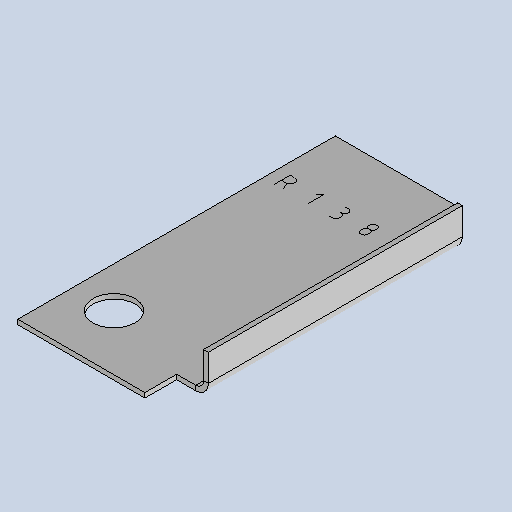
# Autodesk Inventor part: Part14
Saved by Autodesk Inventor 2025.3 (Build 293356030, 356C)
## iProperties
Created: 2026-01-14
Part Number: Part14
Material: Stainless Steel
Document SubType Name: Sheet Metal
Designer: admin
Mass: 447.548 g
Surface Area: 393.455 cm^2
Volume: 55.9434 cm^3
Density: 8 g/cm^3
Flat Pattern Width: 11.8927 cm
Flat Pattern Length: 20 cm
Flat Pattern Area: 237.855 cm^2
Sheet Metal Rule: AISI304 3mm Die 32
Sheet Metal Width: 118,927 mm
Sheet Metal Length: 200,000 mm
Sheet Metal Area: 23785,487 mm^2
Appearance: Default
Author: admin
Autodesk Inventor part; units mm, degrees
ref_plane "YZ Plane" through (0, 0, 0) normal (1, 0, 0) x (0, 1, 0)
ref_plane "XZ Plane" through (0, 0, 0) normal (0, 1, 0) x (-1, 0, 0)
ref_plane "XY Plane" through (0, 0, 0) normal (0, 0, 1) x (1, 0, 0)
sketch "Sketch7" plane through (0, 0, 0) normal (0, 0, 1) x (1, 0, 0)
  line L0 (0, 0) -> (100, 0)
  line L1 (100, 0) -> (100, -200)
  line L2 (100, -200) -> (0, -200)
  line L3 (0, -200) -> (0, 0)
  line L4 (100, 0) -> (80, 0)
  line L5 (80, 0) -> (80, -20)
  line L6 (80, -20) -> (100, -20)
  line L7 (100, -20) -> (100, 0)
  line L8 (100, -200) -> (80, -200)
  line L9 (80, -200) -> (80, -180)
  line L10 (80, -180) -> (100, -180)
  line L11 (100, -180) -> (100, -200)
  dimension "d23" = 100
  dimension "d24" = 200
  dimension "d25" = 20
  dimension "d26" = 20
  measures "d23" distance of L1.end L2.end
  measures "d24" distance of L0.end L1.end
  measures "d25" distance of L6.end L5.end
  measures "d26" distance of L5.end L4.end
extrude "Plate3" add sketch "Sketch7" along normal blind 3 contours L0 L5 L6 L1 L10 L9 L2 L3
sketch "Sketch8" plane through (0, 0, 3) normal (0, 0, 1) x (1, 0, 0)
  line L0 (6.2166, -35.2952) -> (70.6562, -35.2952) construction
  line L1 (70.6562, -35.2952) -> (70.6562, -48.8117) construction
  line L2 (70.6562, -48.8117) -> (6.2166, -48.8117) construction
  line L3 (6.2166, -48.8117) -> (6.2166, -35.2952) construction
  point P0 (0, 0)
  constraints: 2 other
mark "Mark2"
sketch "Sketch9" plane through (0, -200, 3) normal (0, 0, 1) x (1, 0, 0)
  circle A0 centre (25.6213, 34.9394) radius 13.2577
  point P0 (0, 200)
  constraints: 1 centre point
extrude "Cut1" cut sketch "Sketch9" against normal blind 3
sketch "Sketch10" plane through (0, 0, 0) normal (0, 0, -1) x (-1, 0, 0)
  line L0 (-87.8036, -108.5191) -> (-55.956, -108.5191) construction
  line L1 (-55.956, -108.5191) -> (-55.956, -118.5191) construction
  line L2 (-55.956, -118.5191) -> (-87.8036, -118.5191) construction
  line L3 (-87.8036, -118.5191) -> (-87.8036, -108.5191) construction
  point P0 (0, 0)
  constraints: 2 other
mark "Mark3"
sketch "Sketch11" plane through (97, -20, 0) normal (1, 0, 0) x (0, 1, 0)
  line L0 (-160, 0) -> (0, 0)
  line L1 (0, 0) -> (0, 25)
  line L2 (0, 25) -> (-160, 25)
  line L3 (-160, 25) -> (-160, 0)
  constraints: 6 end point, 1 horizontal, 1 perpendicular, 1 vertical
edge flange "Flange2" height 25 angle 90 thickness 3 bend radius 5 thickness toward (1, 0, 0) relief round relief width 3 relief depth 1.5 edges at (100, -100, 3) wall of the first edge with corners at (97, -180, 0) (97, -20, 0) (97, -20, 25) (97, -180, 25)
bend "Bend2"
corner "Corner2"
equation "\"d28\" = Thickness"
equation "\"d27\" = Thickness"
equation "\"d30\" = BendReliefWidth"
equation "\"d31\" = BendReliefDepth"
equation "\"d32\" = MinimumRemnant"
equation "\"d33\" = TransitionRadius"
equation "\"d36\" = BendRadius"
equation "\"d37\" = CornerReliefSize"
equation "\"d38\" = GapSize"
equation "\"d39\" = JacobiRadiusSize"
equation "\"BendReliefWidth\" = Thickness"
equation "\"BendReliefDepth\" = 0.5 * Thickness"
equation "\"CornerReliefSize\" = 4 * Thickness"
equation "\"MinimumRemnant\" = 2 * Thickness"
equation "\"TransitionRadius\" = BendRadius"
equation "\"JacobiRadiusSize\" = BendRadius"
equation "\"GapSize\" = Thickness"
equation "\"Thickness\" = 3"
equation "\"BendRadius\" = 5"
body "Solid2"
